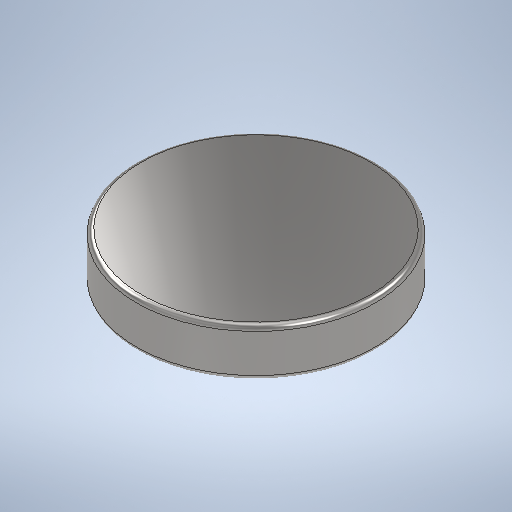
# Autodesk Inventor part: Generic Neodynium Magnet 10mm diameter 2mm height
Saved by Autodesk Inventor 2025.2 (Build 292293000, 293)
## iProperties
Created: 2025-04-15
Part Number: Generic Neodynium Magnet 10mm diameter 2mm height
Material: Steel, Alloy
Document SubType Name: Modeling
Designer: ckyiu
Density: 7.73 g/cm^3
Appearance: Semi-Polished
Author: ckyiu
Autodesk Inventor part; units mm, degrees
ref_plane "YZ Plane" through (0, 0, 0) normal (1, 0, 0) x (0, 1, 0)
ref_plane "XZ Plane" through (0, 0, 0) normal (0, 1, 0) x (-1, 0, 0)
ref_plane "XY Plane" through (0, 0, 0) normal (0, 0, 1) x (1, 0, 0)
sketch "Sketch1" plane through (0, 0, 0) normal (0, 1, 0) x (-1, 0, 0)
  circle A0 centre (0, 0) radius 5
  dimension "d0" = 10
  constraints: 1 centre point, 1 coincident
  measures "d0" diameter of A0
extrude "Extrusion1" add sketch "Sketch1" along normal blind 2
fillet "Fillet1" radius 0.2 2 edges at (5, 0, 0) (5, 2, 0)
